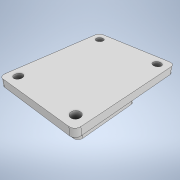
# Autodesk Inventor part: gravity-pcb-mount
Saved by Autodesk Inventor 2020.1 (Build 241239000, 239)
## iProperties
Created: 2019-11-14
Part Number: gravity-pcb-mount
Material: Generic
Document SubType Name: Modeling
Designer: njk024
Density: 1 g/cm^3
Appearance: Default
Author: njk024
Autodesk Inventor part; units mm, degrees
ref_plane "YZ Plane" through (0, 0, 0) normal (1, 0, 0) x (0, 1, 0)
ref_plane "XZ Plane" through (0, 0, 0) normal (0, 1, 0) x (-1, 0, 0)
ref_plane "XY Plane" through (0, 0, 0) normal (0, 0, 1) x (1, 0, 0)
sketch "Sketch1" plane through (0, 0, 0) normal (0, 1, 0) x (-1, 0, 0)
  circle A0 centre (0, 0) radius 1.65
  circle A1 centre (0, -35) radius 1.65
  circle A2 centre (-25, 0) radius 1.65
  circle A3 centre (-25, -35) radius 1.65
  line L0 (0, 0) -> (-25, 0) construction
  line L1 (-25, 0) -> (-25, -35) construction
  line L2 (-25, -35) -> (0, -35) construction
  line L3 (0, -35) -> (0, 0) construction
  line L4 (4, 4) -> (-29, 4)
  line L5 (-29, 4) -> (-29, -39)
  line L6 (-29, -39) -> (4, -39)
  line L7 (4, -39) -> (4, 4)
  dimension "d1" = 3.3
  dimension "d2" = 3.3
  dimension "d4" = 3.3
  dimension "d5" = 3.3
  dimension "d6" = 35
  dimension "d7" = 25
  dimension "d8" = 4
  constraints: 16 end point, 4 centre point, 4 parallel, 2 perpendicular, 1 coincident, 1 horizontal, 3 other
  measures "d1" diameter of A0
  measures "d2" diameter of A1
  measures "d4" diameter of A2
  measures "d5" diameter of A3
  measures "d6" distance of L2.end L0.start
  measures "d7" distance of L0.start L0.end
  measures "d8" distance between parallel lines of L4 L0
extrude "Extrusion1" add sketch "Sketch1" along normal blind 3
sketch "Sketch2" plane through (0, 0, 0) normal (0, -1, 0) x (1, 0, 0)
  circle A0 centre (25, -35) radius 1.65 construction
  circle A1 centre (25, 0) radius 1.65 construction
  circle A2 centre (0, -35) radius 1.65 construction
  circle A3 centre (0, 0) radius 1.65 construction
  line L0 (29, -39) -> (-4, -39) projected
  line L1 (-4, -39) -> (-4, 4) projected
  line L2 (-4, 4) -> (29, 4) projected
  line L3 (29, 4) -> (29, -39) projected
  line L4 (21, -31) -> (4, -31)
  line L5 (4, -31) -> (4, -4)
  line L6 (4, -4) -> (21, -4)
  line L7 (21, -4) -> (21, -31)
  dimension "d11" = 8
  constraints: 8 end point, 3 other
  measures "d11" distance between parallel lines of L3 L7
extrude "Extrusion2" add sketch "Sketch2" along normal blind 12 contours L4 L5 L6 L7
fillet "Fillet1" radius 2 8 edges at (29, 1.5, 4) (-4, 1.5, 4) (-4, 1.5, -39) (29, 1.5, -39) (21, -6, -4) (4, -6, -4) (4, -6, -31) (21, -6, -31)
body "Solid1"
